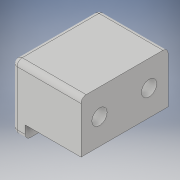
# Autodesk Inventor part: lever-adapter
Saved by Autodesk Inventor 2019 (Build 230136000, 136)
## iProperties
Created: 2021-01-24
Part Number: lever-adapter
Material: Genérico
Document SubType Name: Modeling
Designer: Juan M. Casillas
Density: 1 g/cm^3
Appearance: Valor por defecto
Author: Juan M. Casillas
## iProperties of the stored document lever-adapter_3DPrint.ipt
Created: 2021-01-24
Part Number: lever-adapter_3DPrint
Material: Genérico
Document SubType Name: Modeling
Designer: Juan M. Casillas
Density: 1 g/cm^3
Appearance: Valor por defecto
Author: Juan M. Casillas
Autodesk Inventor part; units mm, degrees
ref_plane "YZ Plane" through (0, 0, 0) normal (1, 0, 0) x (0, 1, 0)
ref_plane "XZ Plane" through (0, 0, 0) normal (0, 1, 0) x (-1, 0, 0)
ref_plane "XY Plane" through (0, 0, 0) normal (0, 0, 1) x (1, 0, 0)
sketch "Sketch1" plane through (0, 0, 0) normal (0, 1, 0) x (-1, 0, 0)
  line L0 (-46, 7.9) -> (16.4908, 7.9)
  line L1 (-46, -7.9) -> (-46, 7.9)
  line L2 (16.4908, -7.9) -> (-46, -7.9)
  line L3 (16.4908, 7.9) -> (16.4908, -7.9)
  circle A0 centre (-27.1464, 0) radius 5.405
  ellipse E0 centre (-40.7943, -4.593) end of major axis (-42.2702, -4.593) minor radius 1.475 construction
  ellipse E1 centre (-40.7943, 5.037) end of major axis (-42.2702, 5.037) minor radius 1.475 construction
  line L4 (-40.7943, -4.593) -> (-35.5886, -4.593) construction
  line L5 (-35.5886, -7.9) -> (-35.5886, 7.9)
  point P0 (0, 0)
  point P1 (0, 0)
  dimension "d0" = 5.2057
  dimension "d1" = 5.2057
  constraints: 12 end point, 2 point on line, 1 centre point, 1 horizontal, 1 perpendicular, 4 other
  measures "d0" distance from line of L1 L4.start
  measures "d1" distance of L4.start L4.end
extrude "Extrusion1" add sketch "Sketch1" along normal blind 10 contours L0 L5 L2 L1
sketch "Sketch2" plane through (46, 0, 7.9) normal (1, 0, 0) x (0, 0, -1)
  line L0 (0, 0) -> (15.8, 0) construction
  line L1 (15.8, 0) -> (15.8, 10) construction
  line L2 (0, 10) -> (15.8, 10) construction
  line L3 (0, 0) -> (0, 10) construction
  line L4 (15.8, 0) -> (15.8, 10) construction
  line L5 (15.8, 5) -> (0, 5) construction
  line L6 (0, 10) -> (15.8, 10) construction
  line L7 (7.9, 10) -> (7.9, 0) construction
  line L8 (12.715, 5) -> (3.085, 5) construction
  circle A0 centre (12.715, 5) radius 1.475
  circle A1 centre (3.085, 5) radius 1.475
  point P0 (7.9, 5)
  dimension "d8" = 9.63
  dimension "d9" = 2.95
  dimension "d10" = 2.95
  dimension "d11" = 5
  constraints: 6 end point, 5 midpoint, 2 centre point, 2 coincident, 1 horizontal, 1 vertical
  measures "d8" distance of L8.start L8.end
  measures "d9" diameter of A0
  measures "d10" diameter of A1
  measures "d11" distance between parallel lines of L0 L5
extrude "Extrusion2" cut sketch "Sketch2" against normal blind 5
thicken "Thicken1" [suppressed]
sketch "Sketch3" plane through (35.5886, 0, 7.9) normal (0, -1, 0) x (1, 0, 0)
  line L0 (10.4114, 0) -> (10.4114, -15.8) construction
  line L1 (0, 0) -> (10.4114, 0) construction
  line L2 (0, -15.8) -> (0, 0) construction
  line L3 (10.4114, -15.8) -> (0, -15.8) construction
  line L4 (10.4114, -11.24) -> (10.4114, -14.19) construction
  line L5 (10.4114, -1.61) -> (10.4114, -4.56) construction
  line L6 (10.4114, -15.8) -> (0, -15.8) construction
  circle A0 centre (3.4114, -12.715) radius 1.45
  circle A1 centre (3.4114, -3.085) radius 1.45
  point P0 (-35.5886, -7.9)
  point P1 (5.2057, -7.9)
  dimension "d17" = 2.9
  dimension "d18" = 2.9
  dimension "d27" = 7
  dimension "d28" = 7
  dimension "d29" = 9.63
  constraints: 2 centre point
  measures "d17" diameter of A0
  measures "d18" diameter of A1
  measures "d27" distance from line of L0 A0.centre
  measures "d28" horizontal distance of A1.centre L5.end
  measures "d29" distance of A1.centre A0.centre
extrude "Extrusion3" cut sketch "Sketch3" against normal blind 7
thicken "Thicken2" operation add thickness 3 both sides no extend neighbours yes toward (-1, 0, 0) faces at (35.5886, 6.6667, -2.6333)
fillet "Fillet2" radius 1 5 edges at (32.5886, 10, 0) (32.5886, 5, 7.9) (32.5886, 5, -7.9) (39.2943, 10, 7.9) (39.2943, 10, -7.9)
thicken "Thicken3" operation add thickness 0.1 both sides no extend neighbours yes toward (0, 0, -1) faces at (41.8629, 3, -7.9)
sketch "Sketch4" plane through (0, 0, 0) normal (0, -1, 0) x (1, 0, 0)
  line L0 (33.5886, 7.9) -> (46, 7.9) projected
  arc A0 (33.5886, 7.9) -> (32.5886, 6.9) centre (33.5886, 6.9) ccw projected
  line L1 (32.5886, -7) -> (32.5886, 6.9) projected
  arc A1 (32.5886, -7) -> (33.5886, -8) centre (33.5886, -7) ccw projected
  line L2 (46, -8) -> (33.5886, -8) projected
  line L3 (35.1886, 7.9) -> (35.1886, -8)
  point P0 (0, 0)
  dimension "d33" = 2.6
  constraints: 2 end point, 2 point on line, 1 perpendicular
  measures "d33" distance between parallel lines of L1 L3
extrude "Extrusion4" add sketch "Sketch4" along normal blind 2.6
fillet "Fillet3" radius 1 5 edges at (32.8815, -2.6, -7.7071) (34.3886, -2.6, -8) (32.8815, -2.6, 7.6071) (34.3886, -2.6, 7.9) (32.5886, -2.6, -0.05)
thicken "Thicken4" operation add thickness 1 both sides no extend neighbours yes toward (0, -1, 0) faces at (41.8629, 10, 2.2667)
thicken "Thicken5" operation add thickness 0.5 both sides no extend neighbours yes toward (0, 0, 1) faces at (38.2591, 5.3333, 7.9)
thicken "Thicken6" operation add thickness 0.5 both sides no extend neighbours yes toward (0, 0, -1) faces at (38.2591, 5.3333, -8)
thicken "Thicken7" operation add thickness 1 both sides no extend neighbours yes toward (0, 1, 0) faces at (41.8629, 9, 2.4333)
equation "\"d1\" = d0"
equation "\"d28\" = d27"
body "Solid1"
